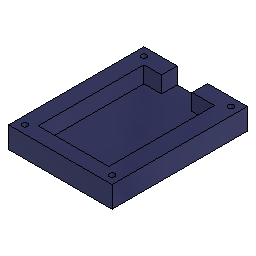
Case (Autodesk Fusion 360 archive; units mm, degrees)
design "Case"
Autodesk Fusion 360 part; units mm, degrees
sketch "Sketch1" plane through (0, 0, 0) normal (0, 0, 1) x (1, 0, 0) in component "Case"
  line L0 (0, 0) -> (42.9, 0)
  line L1 (42.9, 0) -> (42.9, 64.3)
  line L2 (42.9, 64.3) -> (0, 64.3)
  line L3 (0, 64.3) -> (0, 0)
  line L4 (53.4, 73.8) -> (-9.5, 73.8)
  line L5 (-9.5, 73.8) -> (-9.5, -8.5)
  line L6 (-9.5, -8.5) -> (53.4, -8.5)
  line L7 (53.4, -8.5) -> (53.4, 73.8)
  circle A0 centre (-4.5, 68.8) radius 1.7
  circle A1 centre (48.4, 68.8) radius 1.7
  circle A2 centre (48.4, -3.5) radius 1.7
  circle A3 centre (-4.5, -3.5) radius 1.7
  circle A4 centre (48.4, 68.8) radius 3
  circle A5 centre (48.4, -3.5) radius 3
  circle A6 centre (-4.5, 68.8) radius 3
  circle A7 centre (-4.5, -3.5) radius 3
  dimension "d1" = 42.9
  dimension "d2" = 64.3
  dimension "d3" = 62.9
  dimension "d4" = 82.3
  dimension "d5" = 9.5
  dimension "d6" = 9.5
  dimension "d7" = 3.4
  dimension "d8" = 3.4
  dimension "d9" = 3.4
  dimension "d10" = 3.4
  dimension "d11" = 5
  dimension "d12" = 5
  dimension "d13" = 5
  dimension "d14" = 5
  dimension "d15" = 5
  dimension "d16" = 5
  dimension "d17" = 5
  dimension "d18" = 5
  dimension "d19" = 1.3
  dimension "d20" = 1.3
  dimension "d21" = 1.3
  dimension "d22" = 1.3
  constraint horizontal L0
  constraint vertical L1
  constraint horizontal L2
  constraint vertical L3
  constraint coincident L0.start L3.end
  constraint horizontal L4
  constraint vertical L5
  constraint horizontal L6
  constraint vertical L7
  measures "d1" distance of L0.start L0.end
  measures "d2" distance of L0.start L2.end
  measures "d3" distance of L4.start L4.end
  measures "d4" distance of L4.end L5.end
  measures "d5" distance of L2 L4
  measures "d6" distance of L3 L5
  measures "d7" diameter of A0
  measures "d8" diameter of A1
  measures "d9" diameter of A2
  measures "d10" diameter of A3
  measures "d11" distance of L6 A3.centre
  measures "d12" distance of L5 A3.centre
  measures "d13" distance of L6 A2.centre
  measures "d14" distance of L7 A2.centre
  measures "d15" distance of L4 A1.centre
  measures "d16" distance of L7 A1.centre
  measures "d17" distance of L4 A0.centre
  measures "d18" distance of L5 A0.centre
extrude "Extrude1" add sketch "Sketch1" along normal blind 9.9 from surface at 3.1 contours A4 | A5 | A6 | A7 makes body 1 at (51.3963, -3.6495, 9.7) makes body 2 at (50.9599, 70.3643, 9.7) makes body 3 at (-1.5037, -3.6495, 9.7) makes body 4 at (-7.0599, 67.2357, 9.7) in component "Case"
extrude "Extrude2" add sketch "Sketch1" along normal blind 13 contours L4 L5 L6 L7 bodies 1 2 3 4 in component "Case"
extrude "Extrude3" add sketch "Sketch1" along normal blind 3 contours L0 L1 L2 L3 bodies 1 in component "Case"
sketch "Sketch2" plane through (0, 0, 13) normal (0, 0, 1) x (-1, 0, 0) in component "Case"
  circle A0 centre (-48.4, 3.5) radius 1.7
  circle A1 centre (4.5, -68.8) radius 1.7
  line L0 (0, 0) -> (0, -64.3)
  line L1 (0, -64.3) -> (-42.9, -64.3)
  line L2 (-42.9, -64.3) -> (-42.9, 0)
  line L3 (-42.9, 0) -> (0, 0)
  line L4 (-53.4, 8.5) -> (-53.4, -73.8)
  line L5 (-53.4, -73.8) -> (9.5, -73.8)
  line L6 (9.5, -73.8) -> (9.5, 8.5)
  line L7 (9.5, 8.5) -> (-53.4, 8.5)
  circle A2 centre (-48.4, -68.8) radius 1.7
  circle A3 centre (4.5, 3.5) radius 1.7
  line L8 (0, -64.3) -> (0, 0)
  line L9 (0, 0) -> (-42.9, 0)
  line L10 (-42.9, 0) -> (-42.9, -64.3)
  line L11 (-42.9, -64.3) -> (0, -64.3)
  line L12 (-10.71, -73.8) -> (-29.21, -73.8)
  line L13 (-29.21, -73.8) -> (-29.21, -64.3)
  line L14 (-29.21, -64.3) -> (-10.71, -64.3)
  line L15 (-10.71, -64.3) -> (-10.71, -73.8)
  dimension "d31" = 10.71
  dimension "d32" = 13.69
  constraint horizontal L12
  constraint vertical L13
  constraint horizontal L14
  constraint vertical L15
  constraint coincident L1 L13.end
  constraint coincident L5 L12.start
  measures "d31" distance of L0.end L14.end
  measures "d32" distance of L1.end L13.end
extrude "Extrude4" cut sketch "Sketch2" against normal blind 10 contours L1 L5 L11 L12 L13 L14 L15 bodies 1 in component "Case"
component "Case" placed x (1, 0, 0) y (0, 1, 0) z (0, 0, 1) at (0, 0, 0)
equation "d31 = 14.46 mm - 3.75 mm"
equation "d32 = 14.46 mm - 0.77 mm"
named bodies: "Case"
